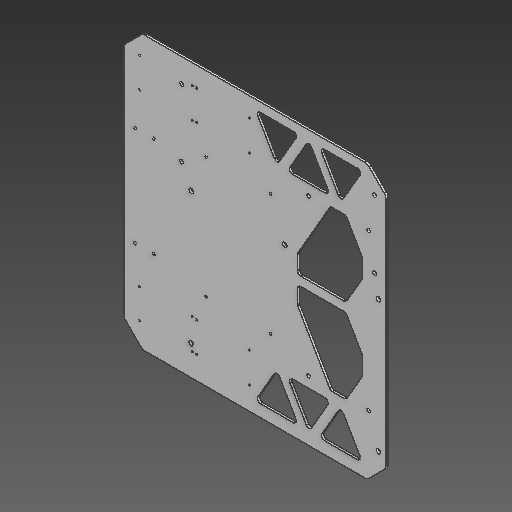
# Autodesk Inventor part: ChestTopPanel
Saved by Autodesk Inventor 2025.2 (Build 292293000, 293)
## iProperties
Created: 2025-10-05
Part Number: ChestTopPanel
Material: Generic
Document SubType Name: Sheet Metal
Designer: valer
Density: 1 g/cm^3
Sheet Metal Rule: Default
Appearance: Default
Author: valer
Autodesk Inventor part; units mm, degrees
ref_plane "YZ Plane" through (0, 0, 0) normal (1, 0, 0) x (0, 1, 0)
ref_plane "XZ Plane" through (0, 0, 0) normal (0, 1, 0) x (-1, 0, 0)
ref_plane "XY Plane" through (0, 0, 0) normal (0, 0, 1) x (1, 0, 0)
sketch "Base" plane through (0, 0, 0) normal (0, 0, 1) x (1, 0, 0)
  line L0 (370.5814, -184.5855) -> (20.5814, -184.5855)
  line L1 (20.5814, -184.5855) -> (20.5814, 180.4145)
  line L2 (20.5814, 180.4145) -> (370.5814, 180.4145)
  line L3 (370.5814, 180.4145) -> (370.5814, -184.5855)
  point P0 (0, 0)
  dimension "d1" = 365
  dimension "d3" = 350
  measures "d1" distance of L2.end L0.start
  measures "d3" distance of L0.start L0.end
extrude "Plate1" add sketch "Base" along normal blind 3
chamfer "BaseChamfersFeature" distance 25 angle 45 4 edges at (20.5814, 180.4145, 1.5) (370.5814, 180.4145, 1.5) (370.5814, -184.5855, 1.5) (20.5814, -184.5855, 1.5)
fillet "BaseFilletsFeature" radius 8 8 edges at (20.5814, 155.4145, 1.5) (45.5814, 180.4145, 1.5) (20.5814, -159.5855, 1.5) (45.5814, -184.5855, 1.5) (345.5814, 180.4145, 1.5) (370.5814, 155.4145, 1.5) (370.5814, -159.5855, 1.5) (345.5814, -184.5855, 1.5)
sketch "ChargerMountHoles" plane through (0, 0, 0) normal (0, 0, -1) x (-1, 0, 0)
  line L0 (-338.5814, 164.0145) -> (-338.5814, 43.4145) construction
  line L1 (-338.5814, 43.4145) -> (-358.8814, 43.4145) construction
  arc A0 (-364.5814, 49.1145) -> (-358.8814, 43.4145) centre (-358.8814, 49.1145) ccw construction
  line L2 (-364.5814, 49.1145) -> (-364.5814, 55.9145) construction
  line L3 (-364.5814, 55.9145) -> (-355.4314, 55.9145) construction
  arc A1 (-355.4314, 55.9145) -> (-355.4314, 61.6145) centre (-355.4314, 58.7645) ccw construction
  line L4 (-355.4314, 61.6145) -> (-364.5814, 61.6145) construction
  line L5 (-364.5814, 61.6145) -> (-364.5814, 145.8145) construction
  line L6 (-364.5814, 145.8145) -> (-355.4314, 145.8145) construction
  arc A2 (-355.4314, 145.8145) -> (-355.4314, 151.5145) centre (-355.4314, 148.6645) ccw construction
  line L7 (-355.4314, 151.5145) -> (-364.5814, 151.5145) construction
  line L8 (-364.5814, 151.5145) -> (-364.5814, 158.3145) construction
  arc A3 (-358.8814, 164.0145) -> (-364.5814, 158.3145) centre (-358.8814, 158.3145) ccw construction
  line L9 (-358.8814, 164.0145) -> (-338.5814, 164.0145) construction
  line L10 (-114.5814, 43.4145) -> (-114.5814, 164.0145) construction
  line L11 (-114.5814, 164.0145) -> (-94.2814, 164.0145) construction
  arc A4 (-88.5814, 158.3145) -> (-94.2814, 164.0145) centre (-94.2814, 158.3145) ccw construction
  line L12 (-88.5814, 158.3145) -> (-88.5814, 151.5145) construction
  line L13 (-88.5814, 151.5145) -> (-97.7314, 151.5145) construction
  arc A5 (-97.7314, 151.5145) -> (-97.7314, 145.8145) centre (-97.7314, 148.6645) ccw construction
  line L14 (-97.7314, 145.8145) -> (-88.5814, 145.8145) construction
  line L15 (-88.5814, 145.8145) -> (-88.5814, 61.6145) construction
  line L16 (-88.5814, 61.6145) -> (-97.7314, 61.6145) construction
  arc A6 (-97.7314, 61.6145) -> (-97.7314, 55.9145) centre (-97.7314, 58.7645) ccw construction
  line L17 (-97.7314, 55.9145) -> (-88.5814, 55.9145) construction
  line L18 (-88.5814, 55.9145) -> (-88.5814, 49.1145) construction
  arc A7 (-94.2814, 43.4145) -> (-88.5814, 49.1145) centre (-94.2814, 49.1145) ccw construction
  line L19 (-94.2814, 43.4145) -> (-114.5814, 43.4145) construction
  circle A8 centre (-97.7314, 58.7645) radius 2.5
  circle A9 centre (-97.7314, 148.6645) radius 2.5
  circle A10 centre (-355.4314, 58.7645) radius 2.5
  circle A11 centre (-355.4314, 148.6645) radius 2.5
  point P0 (0, 0)
  dimension "d14" = 5
  constraints: 4 centre point, 4 coincident, 3 equal radius
  measures "d14" diameter of A8
extrude "ChargerMountHolesFeature" cut sketch "ChargerMountHoles" against normal blind 3
sketch "ShelfMount" plane through (0, 0, 0) normal (0, 0, -1) x (-1, 0, 0)
  circle A0 centre (-360.5814, 31.4145) radius 3
  circle A1 centre (-235.5814, 31.4145) radius 3
  circle A2 centre (-110.5814, 31.4145) radius 3
  circle A3 centre (-235.5814, 31.4145) radius 3
  circle A4 centre (-110.5814, -144.5855) radius 3
  circle A5 centre (-235.5814, -144.5855) radius 3
  circle A6 centre (-360.5814, -144.5855) radius 3
  point P0 (0, 0)
extrude "ShelfMountFeature" cut sketch "ShelfMount" against normal blind 3
sketch "TopElectricalMountHoles" plane through (0, 0, 0) normal (0, 0, -1) x (-1, 0, 0)
  arc A0 (-270.2879, 102.25) -> (-264.5748, 102.25) centre (-267.4314, 104) ccw construction
  arc A1 (-350.2879, 102.25) -> (-344.5748, 102.25) centre (-347.4314, 104) ccw construction
  arc A2 (-270.2879, -105.75) -> (-264.5748, -105.75) centre (-267.4314, -104) ccw construction
  arc A3 (-350.2879, -105.75) -> (-344.5748, -105.75) centre (-347.4314, -104) ccw construction
  circle A4 centre (-35.5814, 66.75) radius 2.25 construction
  circle A5 centre (-60.5814, 66.75) radius 2.25 construction
  circle A6 centre (-60.5814, -66.75) radius 2.25 construction
  circle A7 centre (-35.5814, -66.75) radius 2.25 construction
  circle A8 centre (-41.5814, 153.562) radius 1.25 projected
  circle A9 centre (-41.5814, 113.8591) radius 1.25 projected
  circle A10 centre (-111.7916, 153.9785) radius 1.25 projected
  circle A11 centre (-111.7916, 113.4426) radius 1.25 projected
  circle A12 centre (-117.7916, 153.9785) radius 1.25 projected
  circle A13 centre (-117.7916, 114.2755) radius 1.25 projected
  circle A14 centre (-188.0018, 154.3949) radius 1.25 projected
  circle A15 centre (-188.0018, 113.8591) radius 1.25 projected
  line L0 (74.1163, 0) -> (-444.6976, 0) construction
  circle A16 centre (-41.5814, -153.562) radius 1.25
  circle A17 centre (-41.5814, -113.8591) radius 1.25
  circle A18 centre (-111.7916, -153.9785) radius 1.25
  circle A19 centre (-111.7916, -113.4426) radius 1.25
  circle A20 centre (-117.7916, -153.9785) radius 1.25
  circle A21 centre (-117.7916, -114.2755) radius 1.25
  circle A22 centre (-188.0018, -154.3949) radius 1.25
  circle A23 centre (-188.0018, -113.8591) radius 1.25
  circle A24 centre (-130.4314, 80.875) radius 1.6 projected
  circle A25 centre (-216.5814, 80.875) radius 1.6 projected
  circle A26 centre (-216.5814, -80.875) radius 1.6 projected
  circle A27 centre (-130.4314, -80.875) radius 1.6 projected
  circle A28 centre (-267.4314, 104) radius 2.25
  circle A29 centre (-347.4314, 104) radius 2.25
  circle A30 centre (-267.4314, -104) radius 2.25
  circle A31 centre (-347.4314, -104) radius 2.25
  circle A32 centre (-35.5814, 66.75) radius 1.75
  circle A33 centre (-60.5814, 66.75) radius 1.75
  circle A34 centre (-60.5814, -66.75) radius 1.75
  circle A35 centre (-35.5814, -66.75) radius 1.75
  point P0 (0, 0)
  dimension "d31" = 3.35
  dimension "d32" = 4.5
  dimension "d33" = 4.5
  dimension "d34" = 4.5
  dimension "d35" = 4.5
  dimension "d36" = 3.5
  constraints: 16 centre point, 8 coincident, 8 symmetric about line, 3 equal radius, 8 other
  measures "d31" radius of A0
  measures "d32" diameter of A28
  measures "d33" diameter of A29
  measures "d34" diameter of A30
  measures "d35" diameter of A31
  measures "d36" diameter of A32
extrude "TopMountHolesFeature" cut sketch "TopElectricalMountHoles" against normal blind 3
sketch "TopCuts" plane through (0, 0, 0) normal (0, 0, -1) x (-1, 0, 0)
  line L0 (-196.1462, 168.4145) -> (-253.8813, 168.4145)
  line L1 (-253.8813, 168.4145) -> (-225.0138, 118.4145)
  line L2 (-225.0138, 118.4145) -> (-196.1462, 168.4145)
  line L3 (-238.8702, 118.4145) -> (-267.7377, 168.4145)
  line L4 (-267.7377, 168.4145) -> (-296.6052, 118.4145)
  line L5 (-296.6052, 118.4145) -> (-238.8702, 118.4145)
  line L6 (-281.5941, 168.4145) -> (-310.4616, 118.4145)
  line L7 (-310.4616, 118.4145) -> (-339.3291, 168.4145)
  line L8 (-339.3291, 168.4145) -> (-281.5941, 168.4145)
  line L9 (-342.2676, 180.4145) -> (-48.8951, 180.4145) projected
  line L10 (-225.0138, 118.4145) -> (-310.4616, 118.4145) construction
  line L11 (-253.8813, 168.4145) -> (-281.5941, 168.4145) construction
  arc A0 (-342.2676, 180.4145) -> (-347.9245, 178.0713) centre (-342.2676, 172.4145) ccw projected
  line L12 (74.1163, 0) -> (-444.6976, 0) construction
  line L13 (-196.1462, -168.4145) -> (-253.8813, -168.4145)
  line L14 (-253.8813, -168.4145) -> (-225.0138, -118.4145)
  line L15 (-225.0138, -118.4145) -> (-196.1462, -168.4145)
  line L16 (-238.8702, -118.4145) -> (-267.7377, -168.4145)
  line L17 (-267.7377, -168.4145) -> (-296.6052, -118.4145)
  line L18 (-296.6052, -118.4145) -> (-238.8702, -118.4145)
  line L19 (-281.5941, -168.4145) -> (-310.4616, -118.4145)
  line L20 (-310.4616, -118.4145) -> (-339.3291, -168.4145)
  line L21 (-339.3291, -168.4145) -> (-281.5941, -168.4145)
  line L22 (-317.3898, 106.4145) -> (-339.3291, 68.4145)
  line L23 (-317.3898, 106.4145) -> (-296.6052, 106.4145)
  line L24 (-296.6052, 106.4145) -> (-252.4873, 30)
  line L25 (-339.3291, 68.4145) -> (-339.3291, 44.4145)
  line L26 (-339.3291, 44.4145) -> (-317.1505, 6)
  line L27 (-317.1505, 6) -> (-252.4873, 6)
  line L28 (-252.4873, 30) -> (-252.4873, 6)
  line L29 (-339.3291, 168.4145) -> (-339.3291, 68.4145) construction
  line L30 (-296.6052, 118.4145) -> (-296.6052, 106.4145) construction
  line L31 (-317.3898, -106.4145) -> (-339.3291, -68.4145)
  line L32 (-317.3898, -106.4145) -> (-296.6052, -106.4145)
  line L33 (-296.6052, -106.4145) -> (-252.4873, -30)
  line L34 (-339.3291, -68.4145) -> (-339.3291, -44.4145)
  line L35 (-339.3291, -44.4145) -> (-317.1505, -6)
  line L36 (-317.1505, -6) -> (-252.4873, -6)
  line L37 (-252.4873, -30) -> (-252.4873, -6)
  point P0 (0, 0)
  point P1 (-345.3291, 179.8055)
  dimension "d39" = 60
  dimension "d40" = 60
  dimension "d41" = 60
  dimension "d42" = 60
  dimension "d43" = 12
  dimension "d44" = 12
  dimension "d45" = 6
  dimension "d46" = 62
  dimension "d47" = 12
  dimension "d48" = 120
  dimension "d49" = 24
  dimension "d50" = 24
  dimension "d51" = 6
  constraints: 74 end point, 16 symmetric about line, 5 parallel, 3 collinear, 3 horizontal, 3 perpendicular, 3 point on line, 1 midpoint, 1 point on circle, 1 vertical
  measures "d39" angle of L0 L2
  measures "d40" angle of L1 L0
  measures "d41" angle of L6 L8
  measures "d42" angle of L7 L8
  measures "d43" distance between parallel lines of L3 L1
  measures "d44" distance between parallel lines of L9 L0
  measures "d45" horizontal distance of point (-345.329, 179.806) L7.end
  measures "d46" distance between parallel lines of L9 L10
  measures "d47" distance between parallel lines of L23 L5
  measures "d48" angle of L24 L23
  measures "d49" distance of L22.end L25.end
  measures "d50" distance of L24.end L27.end
  measures "d51" distance between parallel lines of L12 L27
extrude "TopCutsFeature" cut sketch "TopCuts" against normal blind 3
fillet "TopCutFilletsFeature" radius 4 31 edges at (196.1462, 168.4145, 1.5) (253.8813, 168.4145, 1.5) (225.0138, 118.4145, 1.5) (238.8702, 118.4145, 1.5) (267.7377, 168.4145, 1.5) (296.6052, 118.4145, 1.5) (281.5941, 168.4145, 1.5) (310.4616, 118.4145, 1.5) (339.3291, 168.4145, 1.5) (296.6052, 106.4145, 1.5) (317.3898, 106.4145, 1.5) (252.4873, 30, 1.5) (252.4873, 6, 1.5) (317.1505, 6, 1.5) (339.3291, 68.4145, 1.5) (317.1505, -6, 1.5) (252.4873, -6, 1.5) (252.4873, -30, 1.5) (339.3291, -44.4145, 1.5) (339.3291, -68.4145, 1.5) (317.3898, -106.4145, 1.5) (296.6052, -106.4145, 1.5) (310.4616, -118.4145, 1.5) (339.3291, -168.4145, 1.5) (281.5941, -168.4145, 1.5) (267.7377, -168.4145, 1.5) (296.6052, -118.4145, 1.5) (238.8702, -118.4145, 1.5) (225.0138, -118.4145, 1.5) (196.1462, -168.4145, 1.5) (253.8813, -168.4145, 1.5)
equation "\"d15\" = Thickness"
equation "\"d29\" = Thickness"
equation "\"d37\" = Thickness"
equation "\"d52\" = Thickness"
equation "\"d4\" = Thickness"
equation "\"BendRadius\" = Thickness"
equation "\"BendReliefWidth\" = Thickness"
equation "\"BendReliefDepth\" = 0.5 * Thickness"
equation "\"CornerReliefSize\" = 4 * Thickness"
equation "\"MinimumRemnant\" = 2 * Thickness"
equation "\"TransitionRadius\" = BendRadius"
equation "\"JacobiRadiusSize\" = BendRadius"
equation "\"GapSize\" = Thickness"
equation "\"Thickness\" = 3"
body "Solid1"
